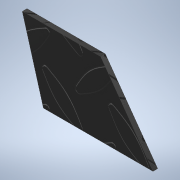
# Autodesk Inventor part: Canard Fin
Saved by Autodesk Inventor 2020 (Build 240168000, 168)
## iProperties
Created: 2022-11-08
Part Number: Canard Fin
Material: FibreGlass
Document SubType Name: Modeling
Designer: Hp
Density: 1500 g/cm^3
Appearance: Diamond plate 2 - Dark Gray
Author: Hp
Autodesk Inventor part; units mm, degrees
ref_plane "YZ Plane" through (0, 0, 0) normal (1, 0, 0) x (0, 1, 0)
ref_plane "XZ Plane" through (0, 0, 0) normal (0, 1, 0) x (-1, 0, 0)
ref_plane "XY Plane" through (0, 0, 0) normal (0, 0, 1) x (1, 0, 0)
sketch "Sketch1" plane through (0, 0, 0) normal (0, 0, 1) x (1, 0, 0)
  line L0 (0, 0) -> (70, 0)
  line L1 (70, 0) -> (36.5279, 46.7533)
  line L2 (36.5279, 46.7533) -> (-13.4721, 46.7533)
  line L3 (-13.4721, 46.7533) -> (0, 0)
  dimension "d0" = 70
  dimension "d1" = 57.5
  dimension "d2" = 54.4
  dimension "d3" = 50
  constraints: 8 end point, 1 horizontal, 1 parallel
  measures "d0" distance of L0.start L0.end
  measures "d1" distance of L0.end L1.end
  measures "d2" angle of L1 L0
  measures "d3" distance of L1.end L2.end
extrude "Extrusion1" add sketch "Sketch1" along normal blind 3
body "Solid1"
